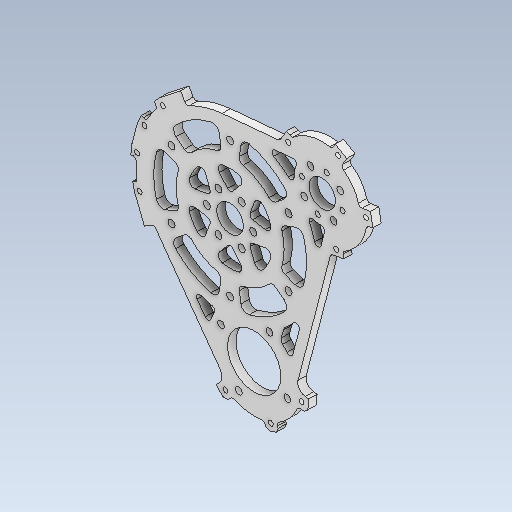
# Autodesk Inventor part: motor_h_1
Saved by Autodesk Inventor 2020 (Build 240168000, 168)
## iProperties
Created: 2020-07-14
Part Number: motor_h_1
Material: ABS Plastic
Document SubType Name: Modeling
Designer: psrobotics
Density: 1.06 g/cm^3
Appearance: Smooth - White
Author: psrobotics
Autodesk Inventor part; units mm, degrees
(part 1 of 3)
ref_plane "YZ Plane" through (0, 0, 0) normal (1, 0, 0) x (0, 1, 0)
ref_plane "XZ Plane" through (0, 0, 0) normal (0, 1, 0) x (-1, 0, 0)
ref_plane "XY Plane" through (0, 0, 0) normal (0, 0, 1) x (1, 0, 0)
sketch "Sketch1" plane through (0, 0, 0) normal (0, 0, 1) x (1, 0, 0)
  circle A0 centre (13.3039, -43.7854) radius 2.1 projected
  circle A1 centre (31.1494, -18.2994) radius 2.1 projected
  line L0 (8.7569, -41.0332) -> (9.9725, -47.9268) projected
  line L1 (12.5142, -47.4787) -> (9.9725, -47.9268) projected
  line L2 (17.8509, -46.5376) -> (12.5142, -47.4787) projected
  line L3 (17.2063, -42.8816) -> (17.8509, -46.5376) projected
  arc A2 (17.2063, -42.8816) -> (25.3756, -36.4162) centre (4.8498, -18.875) ccw projected
  arc A3 (25.3756, -36.4162) -> (28.3534, -32.1635) centre (4.8498, -18.875) ccw projected
  arc A4 (28.3534, -32.1635) -> (31.6348, -22.2755) centre (4.8498, -18.875) ccw projected
  line L4 (31.6348, -22.2755) -> (35.2909, -21.6308) projected
  line L5 (35.2909, -21.6308) -> (34.3498, -16.2941) projected
  line L6 (34.3498, -16.2941) -> (33.9017, -13.7524) projected
  line L7 (33.9017, -13.7524) -> (27.008, -14.9679) projected
  arc A5 (8.7569, -41.0332) -> (27.008, -14.9679) centre (4.8498, -18.875) ccw projected
  circle A6 centre (14.3857, 5.6417) radius 2.1 projected
  circle A7 centre (-15.6668, -2.4109) radius 2.1 projected
  line L8 (16.0998, 0.6106) -> (19.5998, 6.6727) projected
  line L9 (17.3647, 7.9632) -> (19.5998, 6.6727) projected
  line L10 (12.6716, 10.6727) -> (17.3647, 7.9632) projected
  line L11 (10.8154, 7.4577) -> (12.6716, 10.6727) projected
  arc A8 (10.8154, 7.4577) -> (0.4014, 7.756) centre (4.8498, -18.875) ccw projected
  arc A9 (0.4014, 7.756) -> (-4.6132, 6.4123) centre (4.8498, -18.875) ccw projected
  arc A10 (-4.6132, 6.4123) -> (-13.4829, 0.947) centre (4.8498, -18.875) ccw projected
  line L12 (-13.4829, 0.947) -> (-16.6979, 2.8032) projected
  line L13 (-16.6979, 2.8032) -> (-19.4075, -1.8899) projected
  line L14 (-19.4075, -1.8899) -> (-20.6979, -4.125) projected
  line L15 (-20.6979, -4.125) -> (-14.6357, -7.625) projected
  arc A11 (16.0998, 0.6106) -> (-14.6357, -7.625) centre (4.8498, -18.875) ccw projected
  circle A12 centre (-102.1649, -37.0532) radius 2.05 projected
  circle A13 centre (-91.1309, -21.0881) radius 2.05 projected
  circle A14 centre (-106.5395, -53.3794) radius 2.05 projected
  circle A15 centre (-104.9663, -72.7226) radius 2.05 projected
  line L16 (-76.835, -14.1568) -> (-80.3713, -8.0318) projected
  line L17 (-92.9509, -17.9357) -> (-80.3713, -8.0318) projected
  arc A16 (-92.9509, -17.9357) -> (-96.423, -21.7867) centre (-50.585, -59.6232) ccw projected
  line L18 (-95.6743, -22.4047) -> (-96.423, -21.7867) projected
  arc A17 (-95.3624, -25.1669) -> (-95.6743, -22.4047) centre (-96.9475, -23.9472) ccw projected
  arc A18 (-95.3624, -25.1669) -> (-100.1355, -32.4754) centre (-50.585, -59.6232) ccw projected
  arc A19 (-102.79, -33.3003) -> (-100.1355, -32.4754) centre (-101.8895, -31.5145) ccw projected
  line L19 (-103.9829, -32.6988) -> (-102.79, -33.3003) projected
  arc A20 (-103.9829, -32.6988) -> (-106.5047, -38.4279) centre (-50.585, -59.6232) ccw projected
  line L20 (-106.5047, -38.4279) -> (-109.6106, -50.019) projected
  arc A21 (-109.6106, -50.019) -> (-110.2911, -56.2415) centre (-50.585, -59.6232) ccw projected
  line L21 (-110.2911, -56.2415) -> (-108.9573, -56.317) projected
  arc A22 (-107.0709, -58.3586) -> (-108.9573, -56.317) centre (-109.0704, -58.3138) ccw projected
  arc A23 (-107.0709, -58.3586) -> (-106.5915, -67.0745) centre (-50.585, -59.6232) ccw projected
  arc A24 (-108.2427, -69.3107) -> (-106.5915, -67.0745) centre (-108.5741, -67.3383) ccw projected
  line L22 (-108.2427, -69.3107) -> (-109.2001, -69.4715) projected
  arc A25 (-109.2001, -69.4715) -> (-108.1187, -74.5427) centre (-50.585, -59.6232) ccw projected
  line L23 (-108.1187, -74.5427) -> (-102.1764, -89.4094) projected
  line L24 (-102.1764, -89.4094) -> (-96.0514, -85.8732) projected
  arc A26 (-76.835, -14.1568) -> (-96.0514, -85.8732) centre (-50.585, -59.6232) ccw projected
  line L25 (-21.6241, -154.5886) -> (-22.8103, -157.1563) projected
  line L26 (-21.6241, -154.5886) -> (-22.0027, -153.56) projected
  arc A27 (-21.1722, -151.1649) -> (-22.0027, -153.56) centre (-20.1257, -152.8693) ccw projected
  arc A28 (-21.1722, -151.1649) -> (-16.425, -147.5113) centre (-36.0848, -126.8778) ccw projected
  arc A29 (-16.425, -147.5113) -> (-12.2385, -142.4856) centre (-36.0848, -126.8778) ccw projected
  arc A30 (-12.2385, -142.4856) -> (-10.1895, -138.7808) centre (-36.0848, -126.8778) ccw projected
  arc A31 (-8.179, -137.6255) -> (-10.1895, -138.7808) centre (-8.3723, -139.6161) ccw projected
  line L27 (-8.179, -137.6255) -> (-6.0033, -137.8368) projected
  line L28 (-3.8193, -136.0394) -> (-6.0033, -137.8368) projected
  line L29 (-3.8193, -136.0394) -> (-3.2394, -130.0675) projected
  line L30 (-11.2019, -129.2943) -> (-3.2394, -130.0675) projected
  arc A32 (-53.4647, -144.8483) -> (-11.2019, -129.2943) centre (-36.0848, -126.8778) ccw projected
  line L31 (-53.4647, -144.8483) -> (-59.0263, -150.5988) projected
  line L32 (-59.0263, -150.5988) -> (-54.7134, -154.77) projected
  line L33 (-51.8854, -154.7228) -> (-54.7134, -154.77) projected
  line L34 (-51.8854, -154.7228) -> (-50.3657, -153.1515) projected
  arc A33 (-48.0859, -152.7278) -> (-50.3657, -153.1515) centre (-48.9281, -154.5419) ccw projected
  arc A34 (-48.0859, -152.7278) -> (-44.1241, -154.2204) centre (-36.0848, -126.8778) ccw projected
  arc A35 (-44.1241, -154.2204) -> (-37.6784, -155.3332) centre (-36.0848, -126.8778) ccw projected
  arc A36 (-37.6784, -155.3332) -> (-31.6953, -155.0377) centre (-36.0848, -126.8778) ccw projected
  arc A37 (-29.5104, -156.3231) -> (-31.6953, -155.0377) centre (-31.3873, -157.0139) ccw projected
  line L35 (-29.5104, -156.3231) -> (-29.1318, -157.3516) projected
  line L36 (-26.5641, -158.5378) -> (-29.1318, -157.3516) projected
  line L37 (-26.5641, -158.5378) -> (-22.8103, -157.1563) projected
  circle A38 centre (-53.3702, -150.5044) radius 2.05 projected
  circle A39 centre (-26.0687, -154.0932) radius 2.05 projected
  circle A40 centre (-7.6073, -133.6622) radius 2.05 projected
  circle A41 centre (4.8498, -18.875) radius 22.5
  circle A42 centre (-50.585, -59.6232) radius 52.5
  circle A43 centre (-36.0848, -126.8778) radius 25
  circle A44 centre (14.3857, 5.6417) radius 2.1 projected
  line L38 (-50.585, -59.6232) -> (-93.2051, -90.2791)
  line L39 (-36.0848, -126.8778) -> (-56.3801, -141.4758)
  line L40 (-56.3801, -141.4758) -> (-93.2051, -90.2791)
  line L41 (-50.585, -59.6232) -> (-55.4348, -7.3477)
  line L42 (-55.4348, -7.3477) -> (-20.6979, -4.125)
  line L43 (-11.2019, -129.2943) -> (9.9725, -47.9268)
  point P0 (0, 0)
  dimension "d2" = 50
  dimension "d0" = 45
  dimension "d1" = 105
  constraints: 12 end point, 3 coincident, 3 perpendicular, 2 centre point, 2 point on circle, 3 other
  measures "d0" diameter of A41
  measures "d1" diameter of A42
extrude "Extrusion4" add sketch "Sketch1" along normal blind 5 contours A0 | A1 | A5 L7 L6 L5 L4 A4 A3 A2 L3 L2 L1 L0 | A41 A42 A11 A5 | L0 L43 A43 A42 A41 | A42 A43 L38 L41 A41 | A41 A42 | L30 L29 L28 L27 A31 A30 A29 A28 A27 L26 L25 L37 L36 L35 A37 A36 A35 A34 A33 L34 L33 L32 L31 A32 | A32 A43 A42 | A42 L42 L15 A41 | A11 L15 L14 L13 L12 A10 A9 A8 L11 L10 L9 L8 | L41 L38 A42 A26 | A42 A43 | L40 A42 A43 | A26 L24 L23 A25 L22 A24 A23 A22 L21 A21 L20 A20 L19 A19 A18 A17 L18 A16 L17 L16 | A6 | A7 | A12 | A13 | A14 | A15 | A38 | A39 | A40
sketch "Sketch5" plane through (0, 0, 5) normal (0, 0, 1) x (1, 0, 0)
  circle A0 centre (-26.0687, -154.0932) radius 2.05 projected
  circle A1 centre (-53.3702, -150.5044) radius 2.05 projected
  circle A2 centre (-7.6073, -133.6622) radius 2.05 projected
  circle A3 centre (13.3039, -43.7854) radius 2.1 projected
  circle A4 centre (31.1494, -18.2994) radius 2.1 projected
  circle A5 centre (14.3857, 5.6417) radius 2.1 projected
  circle A6 centre (-15.6668, -2.4109) radius 2.1 projected
  circle A7 centre (-91.1309, -21.0881) radius 2.05 projected
  circle A8 centre (-102.1649, -37.0532) radius 2.05 projected
  circle A9 centre (-106.5395, -53.3794) radius 2.05 projected
  circle A10 centre (-104.9663, -72.7226) radius 2.05 projected
  point P0 (0, 0)
hole "Hole2" at (31.1494, -18.2994, 5) at (13.3039, -43.7854, 5) at (-15.6668, -2.4109, 5) at (14.3857, 5.6417, 5) at (-91.1309, -21.0881, 5) at (-102.1649, -37.0532, 5) at (-106.5395, -53.3794, 5) at (-104.9663, -72.7226, 5) at (-53.3702, -150.5044, 5) at (-26.0687, -154.0932, 5) at (-7.6073, -133.6622, 5) direction (0, 0, -1) diameter 3 depth 17
sketch "Sketch6" plane through (0, 0, 5) normal (0, 0, 1) x (1, 0, 0)
  circle A0 centre (-50.585, -59.6232) radius 50 projected
  circle A1 centre (-50.585, -59.6232) radius 5.075 projected
  circle A2 centre (4.8498, -18.875) radius 4.075 projected
  circle A3 centre (4.8498, -18.875) radius 8
  circle A4 centre (-50.585, -59.6232) radius 8
  point P0 (0, 0)
  dimension "d30" = 16
  dimension "d31" = 16
  constraints: 2 centre point, 2 coincident
  measures "d30" diameter of A3
  measures "d31" diameter of A4
extrude "Extrusion5" cut sketch "Sketch6" against normal blind 5 contours A1 | A2 | A3 | A4
sketch "Sketch7" plane through (0, 0, 5) normal (0, 0, 1) x (1, 0, 0)
  circle A0 centre (-36.0848, -126.8778) radius 17.5 projected
  circle A1 centre (-43.7823, -118.4013) radius 2.075 projected
  circle A2 centre (-28.3873, -135.3543) radius 2.075 projected
  circle A3 centre (-27.6083, -119.1803) radius 2.075 projected
  circle A4 centre (-44.5613, -134.5753) radius 2.075 projected
  circle A5 centre (-36.0848, -126.8778) radius 16
  point P0 (0, 0)
  dimension "d34" = 32
  constraints: 1 centre point, 1 coincident
  measures "d34" diameter of A5
extrude "Extrusion6" cut sketch "Sketch7" against normal blind 5 contours A1 | A2 | A3 | A4 | A5
fillet "Fillet6" radius 5 1 edges at (-11.2019, -129.2943, 2.5)
fillet "Fillet7" radius 6 1 edges at (-53.4647, -144.8483, 2.5)
sketch "Sketch8" plane through (0, 0, 5) normal (0, 0, 1) x (1, 0, 0)
  circle A0 centre (-36.0848, -126.8778) radius 16 projected
  circle A1 centre (-50.585, -59.6232) radius 8 projected
  circle A2 centre (4.8498, -18.875) radius 8 projected
  circle A3 centre (-26.0687, -154.0932) radius 1.5 projected
  circle A4 centre (-104.9663, -72.7226) radius 1.5 projected
  circle A5 centre (-102.1649, -37.0532) radius 1.5 projected
  circle A6 centre (14.3857, 5.6417) radius 1.5 projected
  circle A7 centre (13.3039, -43.7854) radius 1.5 projected
  circle A8 centre (31.1494, -18.2994) radius 1.5 projected
  circle A9 centre (-15.6668, -2.4109) radius 1.5 projected
  circle A10 centre (-91.1309, -21.0881) radius 1.5 projected
  circle A11 centre (-106.5395, -53.3794) radius 1.5 projected
  circle A12 centre (-53.3702, -150.5044) radius 1.5 projected
  circle A13 centre (-7.6073, -133.6622) radius 1.5 projected
  line L0 (-9.7265, -123.6247) -> (9.9725, -47.9268) projected
  line L1 (9.9725, -47.9268) -> (17.8509, -46.5376) projected
  line L2 (17.8509, -46.5376) -> (17.2063, -42.8816) projected
  arc A14 (17.2063, -42.8816) -> (31.6348, -22.2755) centre (4.8498, -18.875) ccw projected
  line L3 (31.6348, -22.2755) -> (35.2909, -21.6308) projected
  line L4 (35.2909, -21.6308) -> (33.9017, -13.7524) projected
  line L5 (33.9017, -13.7524) -> (27.008, -14.9679) projected
  arc A15 (27.008, -14.9679) -> (16.0998, 0.6106) centre (4.8498, -18.875) ccw projected
  line L6 (16.0998, 0.6106) -> (19.5998, 6.6727) projected
  line L7 (19.5998, 6.6727) -> (12.6716, 10.6727) projected
  line L8 (12.6716, 10.6727) -> (10.8154, 7.4577) projected
  arc A16 (10.8154, 7.4577) -> (-13.4829, 0.947) centre (4.8498, -18.875) ccw projected
  line L9 (-13.4829, 0.947) -> (-16.6979, 2.8032) projected
  line L10 (-16.6979, 2.8032) -> (-20.6979, -4.125) projected
  line L11 (-20.6979, -4.125) -> (-55.4348, -7.3477) projected
  arc A17 (-55.4348, -7.3477) -> (-76.835, -14.1568) centre (-50.585, -59.6232) ccw projected
  line L12 (-76.835, -14.1568) -> (-80.3713, -8.0318) projected
  line L13 (-80.3713, -8.0318) -> (-92.9509, -17.9357) projected
  arc A18 (-92.9509, -17.9357) -> (-96.423, -21.7867) centre (-50.585, -59.6232) ccw projected
  line L14 (-96.423, -21.7867) -> (-95.6743, -22.4047) projected
  arc A19 (-95.3624, -25.1669) -> (-95.6743, -22.4047) centre (-96.9475, -23.9472) ccw projected
  arc A20 (-95.3624, -25.1669) -> (-100.1355, -32.4754) centre (-50.585, -59.6232) ccw projected
  arc A21 (-102.79, -33.3003) -> (-100.1355, -32.4754) centre (-101.8895, -31.5145) ccw projected
  line L15 (-102.79, -33.3003) -> (-103.9829, -32.6988) projected
  arc A22 (-103.9829, -32.6988) -> (-106.5047, -38.4279) centre (-50.585, -59.6232) ccw projected
  line L16 (-106.5047, -38.4279) -> (-109.6106, -50.019) projected
  arc A23 (-109.6106, -50.019) -> (-110.2911, -56.2415) centre (-50.585, -59.6232) ccw projected
  line L17 (-110.2911, -56.2415) -> (-108.9573, -56.317) projected
  arc A24 (-107.0709, -58.3586) -> (-108.9573, -56.317) centre (-109.0704, -58.3138) ccw projected
  arc A25 (-107.0709, -58.3586) -> (-106.5915, -67.0745) centre (-50.585, -59.6232) ccw projected
  arc A26 (-108.2427, -69.3107) -> (-106.5915, -67.0745) centre (-108.5741, -67.3383) ccw projected
  line L18 (-108.2427, -69.3107) -> (-109.2001, -69.4715) projected
  arc A27 (-109.2001, -69.4715) -> (-108.1187, -74.5427) centre (-50.585, -59.6232) ccw projected
  line L19 (-108.1187, -74.5427) -> (-102.1764, -89.4094) projected
  line L20 (-102.1764, -89.4094) -> (-96.0514, -85.8732) projected
  arc A28 (-96.0514, -85.8732) -> (-93.2051, -90.2791) centre (-50.585, -59.6232) ccw projected
  line L21 (-93.2051, -90.2791) -> (-56.6733, -141.0681) projected
  arc A29 (-57.2313, -148.7428) -> (-56.6733, -141.0681) centre (-61.5442, -144.5716) ccw projected
  line L22 (-57.2313, -148.7428) -> (-59.0263, -150.5988) projected
  line L23 (-59.0263, -150.5988) -> (-54.7134, -154.77) projected
  line L24 (-54.7134, -154.77) -> (-51.8854, -154.7228) projected
  line L25 (-51.8854, -154.7228) -> (-50.3657, -153.1515) projected
  arc A30 (-48.0859, -152.7278) -> (-50.3657, -153.1515) centre (-48.9281, -154.5419) ccw projected
  arc A31 (-48.0859, -152.7278) -> (-31.6953, -155.0377) centre (-36.0848, -126.8778) ccw projected
  arc A32 (-29.5104, -156.3231) -> (-31.6953, -155.0377) centre (-31.3873, -157.0139) ccw projected
  line L26 (-29.5104, -156.3231) -> (-29.1318, -157.3516) projected
  line L27 (-29.1318, -157.3516) -> (-26.5641, -158.5378) projected
  line L28 (-26.5641, -158.5378) -> (-22.8103, -157.1563) projected
  line L29 (-22.8103, -157.1563) -> (-21.6241, -154.5886) projected
  line L30 (-21.6241, -154.5886) -> (-22.0027, -153.56) projected
  arc A33 (-21.1722, -151.1649) -> (-22.0027, -153.56) centre (-20.1257, -152.8693) ccw projected
  arc A34 (-21.1722, -151.1649) -> (-10.1895, -138.7808) centre (-36.0848, -126.8778) ccw projected
  arc A35 (-8.179, -137.6255) -> (-10.1895, -138.7808) centre (-8.3723, -139.6161) ccw projected
  line L31 (-8.179, -137.6255) -> (-6.0033, -137.8368) projected
  line L32 (-6.0033, -137.8368) -> (-3.8193, -136.0394) projected
  line L33 (-3.8193, -136.0394) -> (-3.2394, -130.0675) projected
  line L34 (-3.2394, -130.0675) -> (-5.371, -129.8605) projected
  arc A36 (-9.7265, -123.6247) -> (-5.371, -129.8605) centre (-4.8877, -124.8839) ccw projected
  circle A37 centre (-50.585, -59.6232) radius 15
  circle A38 centre (-50.585, -59.6232) radius 46
  circle A39 centre (-50.585, -59.6232) radius 32.5
  line L35 (-50.585, -59.6232) -> (3.2809, -73.6408)
  line L36 (-9.7265, -123.6247) -> (9.9725, -47.9268) projected
  line L37 (-50.585, -59.6232) -> (-38.3591, -103.9687)
  circle A40 centre (-50.585, -59.6232) radius 8 projected
  line L38 (-50.585, -59.6232) -> (-11.4, -83.7174)
  line L39 (-50.585, -59.6232) -> (-96.0514, -85.8732)
  line L40 (-50.585, -59.6232) -> (-86.3338, -88.5719)
  line L41 (-50.585, -59.6232) -> (-93.5297, -76.1081)
  line L42 (-50.585, -59.6232) -> (-93.5297, -43.1382)
  point P0 (0, 0)
  point P1 (-80.9264, -47.9762)
  point P2 (-80.9264, -71.2701)
  dimension "d39" = 30
  dimension "d40" = 92
  dimension "d41" = 65
  dimension "d42" = 60
  dimension "d43" = 17
  dimension "d44" = 9
  dimension "d45" = 9
  dimension "d46" = 42
  constraints: 14 end point, 5 point on circle, 3 centre point, 3 coincident, 1 perpendicular, 1 point on line
  measures "d39" diameter of A37
  measures "d40" diameter of A38
  measures "d41" diameter of A39
  measures "d42" angle of L35 L37
  measures "d43" angle of L35 L38
  measures "d44" angle of L39 L40
  measures "d45" angle of L39 L41
  measures "d46" angle of L41 L42
extrude "Extrusion7" cut sketch "Sketch8" against normal blind 10 contours A39 L41 A38 L42
pattern_circular "Circular Pattern1" count 6 over 360 about axis through (-50.585, -59.6232, 5) along (0, 0, -1) of "Extrusion7"
sketch "Sketch9" plane through (0, 0, 5) normal (0, 0, 1) x (1, 0, 0)
  arc A0 (-86.3338, -88.5719) -> (-57.781, -105.0568) centre (-50.585, -59.6232) ccw projected
  line L0 (-86.3338, -88.5719) -> (-75.8423, -80.0761) projected
  arc A1 (-75.8423, -80.0761) -> (-55.6692, -91.723) centre (-50.585, -59.6232) ccw projected
  line L1 (-55.6692, -91.723) -> (-57.781, -105.0568) projected
  arc A2 (-43.3891, -105.0568) -> (-14.8363, -88.5719) centre (-50.585, -59.6232) ccw projected
  line L2 (-43.3891, -105.0568) -> (-45.5009, -91.723) projected
  arc A3 (-45.5009, -91.723) -> (-25.3278, -80.0761) centre (-50.585, -59.6232) ccw projected
  line L3 (-25.3278, -80.0761) -> (-14.8363, -88.5719) projected
  arc A4 (-7.6403, -76.1081) -> (-7.6403, -43.1382) centre (-50.585, -59.6232) ccw projected
  line L4 (-7.6403, -76.1081) -> (-20.2437, -71.2701) projected
  arc A5 (-20.2437, -71.2701) -> (-20.2437, -47.9762) centre (-50.585, -59.6232) ccw projected
  line L5 (-20.2437, -47.9762) -> (-7.6403, -43.1382) projected
  arc A6 (-14.8363, -30.6744) -> (-43.3891, -14.1895) centre (-50.585, -59.6232) ccw projected
  line L6 (-14.8363, -30.6744) -> (-25.3278, -39.1703) projected
  arc A7 (-25.3278, -39.1703) -> (-45.5009, -27.5233) centre (-50.585, -59.6232) ccw projected
  line L7 (-45.5009, -27.5233) -> (-43.3891, -14.1895) projected
  arc A8 (-57.781, -14.1895) -> (-86.3338, -30.6744) centre (-50.585, -59.6232) ccw projected
  line L8 (-57.781, -14.1895) -> (-55.6692, -27.5233) projected
  arc A9 (-55.6692, -27.5233) -> (-75.8423, -39.1703) centre (-50.585, -59.6232) ccw projected
  line L9 (-75.8423, -39.1703) -> (-86.3338, -30.6744) projected
  arc A10 (-93.5297, -43.1382) -> (-93.5297, -76.1081) centre (-50.585, -59.6232) ccw projected
  line L10 (-93.5297, -43.1382) -> (-80.9264, -47.9762) projected
  arc A11 (-80.9264, -47.9762) -> (-80.9264, -71.2701) centre (-50.585, -59.6232) ccw projected
  line L11 (-80.9264, -71.2701) -> (-93.5297, -76.1081) projected
  circle A12 centre (-36.0848, -126.8778) radius 16 projected
  circle A13 centre (-50.585, -59.6232) radius 8 projected
  circle A14 centre (4.8498, -18.875) radius 8 projected
  circle A15 centre (-26.0687, -154.0932) radius 1.5 projected
  circle A16 centre (-104.9663, -72.7226) radius 1.5 projected
  circle A17 centre (-102.1649, -37.0532) radius 1.5 projected
  circle A18 centre (14.3857, 5.6417) radius 1.5 projected
  circle A19 centre (13.3039, -43.7854) radius 1.5 projected
  circle A20 centre (31.1494, -18.2994) radius 1.5 projected
  circle A21 centre (-15.6668, -2.4109) radius 1.5 projected
  circle A22 centre (-91.1309, -21.0881) radius 1.5 projected
  circle A23 centre (-106.5395, -53.3794) radius 1.5 projected
  circle A24 centre (-53.3702, -150.5044) radius 1.5 projected
  circle A25 centre (-7.6073, -133.6622) radius 1.5 projected
  line L12 (-9.7265, -123.6247) -> (9.9725, -47.9268) projected
  line L13 (9.9725, -47.9268) -> (17.8509, -46.5376) projected
  line L14 (17.8509, -46.5376) -> (17.2063, -42.8816) projected
  arc A26 (17.2063, -42.8816) -> (31.6348, -22.2755) centre (4.8498, -18.875) ccw projected
  line L15 (31.6348, -22.2755) -> (35.2909, -21.6308) projected
  line L16 (35.2909, -21.6308) -> (33.9017, -13.7524) projected
  line L17 (33.9017, -13.7524) -> (27.008, -14.9679) projected
  arc A27 (27.008, -14.9679) -> (16.0998, 0.6106) centre (4.8498, -18.875) ccw projected
  line L18 (16.0998, 0.6106) -> (19.5998, 6.6727) projected
  line L19 (19.5998, 6.6727) -> (12.6716, 10.6727) projected
  line L20 (12.6716, 10.6727) -> (10.8154, 7.4577) projected
  arc A28 (10.8154, 7.4577) -> (-13.4829, 0.947) centre (4.8498, -18.875) ccw projected
  line L21 (-13.4829, 0.947) -> (-16.6979, 2.8032) projected
  line L22 (-16.6979, 2.8032) -> (-20.6979, -4.125) projected
  line L23 (-20.6979, -4.125) -> (-55.4348, -7.3477) projected
  arc A29 (-55.4348, -7.3477) -> (-76.835, -14.1568) centre (-50.585, -59.6232) ccw projected
  line L24 (-76.835, -14.1568) -> (-80.3713, -8.0318) projected
  line L25 (-80.3713, -8.0318) -> (-92.9509, -17.9357) projected
  arc A30 (-92.9509, -17.9357) -> (-96.423, -21.7867) centre (-50.585, -59.6232) ccw projected
  line L26 (-96.423, -21.7867) -> (-95.6743, -22.4047) projected
  arc A31 (-95.3624, -25.1669) -> (-95.6743, -22.4047) centre (-96.9475, -23.9472) ccw projected
  arc A32 (-95.3624, -25.1669) -> (-100.1355, -32.4754) centre (-50.585, -59.6232) ccw projected
  arc A33 (-102.79, -33.3003) -> (-100.1355, -32.4754) centre (-101.8895, -31.5145) ccw projected
  line L27 (-102.79, -33.3003) -> (-103.9829, -32.6988) projected
  arc A34 (-103.9829, -32.6988) -> (-106.5047, -38.4279) centre (-50.585, -59.6232) ccw projected
  line L28 (-106.5047, -38.4279) -> (-109.6106, -50.019) projected
  arc A35 (-109.6106, -50.019) -> (-110.2911, -56.2415) centre (-50.585, -59.6232) ccw projected
  line L29 (-110.2911, -56.2415) -> (-108.9573, -56.317) projected
  arc A36 (-107.0709, -58.3586) -> (-108.9573, -56.317) centre (-109.0704, -58.3138) ccw projected
  arc A37 (-107.0709, -58.3586) -> (-106.5915, -67.0745) centre (-50.585, -59.6232) ccw projected
  arc A38 (-108.2427, -69.3107) -> (-106.5915, -67.0745) centre (-108.5741, -67.3383) ccw projected
  line L30 (-108.2427, -69.3107) -> (-109.2001, -69.4715) projected
  arc A39 (-109.2001, -69.4715) -> (-108.1187, -74.5427) centre (-50.585, -59.6232) ccw projected
  line L31 (-108.1187, -74.5427) -> (-102.1764, -89.4094) projected
  line L32 (-102.1764, -89.4094) -> (-96.0514, -85.8732) projected
  arc A40 (-96.0514, -85.8732) -> (-93.2051, -90.2791) centre (-50.585, -59.6232) ccw projected
  line L33 (-93.2051, -90.2791) -> (-56.6733, -141.0681) projected
  arc A41 (-57.2313, -148.7428) -> (-56.6733, -141.0681) centre (-61.5442, -144.5716) ccw projected
  line L34 (-57.2313, -148.7428) -> (-59.0263, -150.5988) projected
  line L35 (-59.0263, -150.5988) -> (-54.7134, -154.77) projected
  line L36 (-54.7134, -154.77) -> (-51.8854, -154.7228) projected
  line L37 (-51.8854, -154.7228) -> (-50.3657, -153.1515) projected
  arc A42 (-48.0859, -152.7278) -> (-50.3657, -153.1515) centre (-48.9281, -154.5419) ccw projected
  arc A43 (-48.0859, -152.7278) -> (-31.6953, -155.0377) centre (-36.0848, -126.8778) ccw projected
  arc A44 (-29.5104, -156.3231) -> (-31.6953, -155.0377) centre (-31.3873, -157.0139) ccw projected
  line L38 (-29.5104, -156.3231) -> (-29.1318, -157.3516) projected
  line L39 (-29.1318, -157.3516) -> (-26.5641, -158.5378) projected
  line L40 (-26.5641, -158.5378) -> (-22.8103, -157.1563) projected
  line L41 (-22.8103, -157.1563) -> (-21.6241, -154.5886) projected
  line L42 (-21.6241, -154.5886) -> (-22.0027, -153.56) projected
  arc A45 (-21.1722, -151.1649) -> (-22.0027, -153.56) centre (-20.1257, -152.8693) ccw projected
  arc A46 (-21.1722, -151.1649) -> (-10.1895, -138.7808) centre (-36.0848, -126.8778) ccw projected
  arc A47 (-8.179, -137.6255) -> (-10.1895, -138.7808) centre (-8.3723, -139.6161) ccw projected
  line L43 (-8.179, -137.6255) -> (-6.0033, -137.8368) projected
  line L44 (-6.0033, -137.8368) -> (-3.8193, -136.0394) projected
  line L45 (-3.8193, -136.0394) -> (-3.2394, -130.0675) projected
  line L46 (-3.2394, -130.0675) -> (-5.371, -129.8605) projected
  arc A48 (-9.7265, -123.6247) -> (-5.371, -129.8605) centre (-4.8877, -124.8839) ccw projected
  circle A49 centre (-50.585, -59.6232) radius 8 projected
  circle A50 centre (-50.585, -59.6232) radius 13
  circle A51 centre (-50.585, -59.6232) radius 26
  line L47 (-25.3278, -39.1703) -> (-20.2437, -47.9762)
  line L48 (-50.585, -59.6232) -> (-22.7857, -43.5732)
  line L49 (-39.3267, -53.1232) -> (-24.8875, -55.6692)
  line L50 (-39.3267, -53.1232) -> (-34.312, -39.3454)
  point P0 (0, 0)
  dimension "d52" = 26
  dimension "d53" = 52
  dimension "d54" = 40
  dimension "d55" = 40
  constraints: 8 end point, 2 coincident, 2 point on circle, 1 centre point, 1 midpoint, 1 point on line, 3 other
  measures "d53" diameter of A51
  measures "d54" angle of L48 L49
  measures "d55" angle of L48 L50
extrude "Extrusion8" cut sketch "Sketch9" against normal blind 10 contours L50 A51 L48 | L48 A51 L49
pattern_circular "Circular Pattern2" count 6 over 360 about axis through (-50.585, -59.6232, 5) along (0, 0, -1) of "Extrusion8"
fillet "Fillet8" radius 3 2 edges at (-34.312, -39.3454, 2.5) (-24.8875, -55.6692, 2.5)
fillet "Fillet9" radius 2 1 edges at (-39.3267, -53.1232, 2.5)
pattern_circular "Circular Pattern3" count 6 over 360 about axis through (-50.585, -59.6232, 5) along (0, 0, -1) of "Fillet8", "Fillet9"
fillet "Fillet10" radius 3 2 edges at (-45.5009, -27.5233, 2.5) (-25.3278, -39.1703, 2.5)
fillet "Fillet11" radius 4 2 edges at (-43.3891, -14.1895, 2.5) (-14.8363, -30.6744, 2.5)
pattern_circular "Circular Pattern4" count 6 over 360 about axis through (-50.585, -59.6232, 5) along (0, 0, -1) of "Fillet10", "Fillet11"
sketch "Sketch10" plane through (0, 0, 5) normal (0, 0, 1) x (1, 0, 0)
  line L0 (-44.13, -38.9303) -> (-49.053, -44.7973) projected
  arc A0 (-52.1171, -44.7973) -> (-49.053, -44.7973) centre (-50.585, -43.5117) ccw projected
  line L1 (-52.1171, -44.7973) -> (-57.0401, -38.9303) projected
  arc A1 (-55.2842, -34.0514) -> (-57.0401, -38.9303) centre (-54.742, -37.0019) ccw projected
  arc A2 (-45.8859, -34.0514) -> (-55.2842, -34.0514) centre (-50.585, -59.6232) ccw projected
  arc A3 (-44.13, -38.9303) -> (-45.8859, -34.0514) centre (-46.4281, -37.0019) ccw projected
  line L2 (-65.2781, -43.6865) -> (-62.6586, -50.8834) projected
  arc A4 (-64.1907, -53.5371) -> (-62.6586, -50.8834) centre (-64.538, -51.5674) ccw projected
  line L3 (-64.1907, -53.5371) -> (-71.7331, -54.867) projected
  arc A5 (-75.0805, -50.9068) -> (-71.7331, -54.867) centre (-72.2541, -51.9126) ccw projected
  arc A6 (-70.3813, -42.7677) -> (-75.0805, -50.9068) centre (-50.585, -59.6232) ccw projected
  arc A7 (-65.2781, -43.6865) -> (-70.3813, -42.7677) centre (-68.0971, -44.7125) ccw projected
  line L4 (-71.7331, -64.3793) -> (-64.1907, -65.7093) projected
  arc A8 (-62.6586, -68.3629) -> (-64.1907, -65.7093) centre (-64.538, -67.6789) ccw projected
  line L5 (-62.6586, -68.3629) -> (-65.2781, -75.5599) projected
  arc A9 (-70.3813, -76.4787) -> (-65.2781, -75.5599) centre (-68.0971, -74.5338) ccw projected
  arc A10 (-75.0805, -68.3395) -> (-70.3813, -76.4787) centre (-50.585, -59.6232) ccw projected
  arc A11 (-71.7331, -64.3793) -> (-75.0805, -68.3395) centre (-72.2541, -67.3338) ccw projected
  line L6 (-57.0401, -80.316) -> (-52.1171, -74.449) projected
  arc A12 (-49.053, -74.449) -> (-52.1171, -74.449) centre (-50.585, -75.7346) ccw projected
  line L7 (-49.053, -74.449) -> (-44.13, -80.316) projected
  arc A13 (-45.8859, -85.195) -> (-44.13, -80.316) centre (-46.4281, -82.2444) ccw projected
  arc A14 (-55.2842, -85.195) -> (-45.8859, -85.195) centre (-50.585, -59.6232) ccw projected
  arc A15 (-57.0401, -80.316) -> (-55.2842, -85.195) centre (-54.742, -82.2444) ccw projected
  line L8 (-35.892, -75.5599) -> (-38.5115, -68.3629) projected
  arc A16 (-36.9794, -65.7093) -> (-38.5115, -68.3629) centre (-36.6321, -67.6789) ccw projected
  line L9 (-36.9794, -65.7093) -> (-29.437, -64.3793) projected
  arc A17 (-26.0896, -68.3395) -> (-29.437, -64.3793) centre (-28.916, -67.3338) ccw projected
  arc A18 (-30.7888, -76.4787) -> (-26.0896, -68.3395) centre (-50.585, -59.6232) ccw projected
  arc A19 (-35.892, -75.5599) -> (-30.7888, -76.4787) centre (-33.073, -74.5338) ccw projected
  line L10 (-29.437, -54.867) -> (-36.9794, -53.5371) projected
  arc A20 (-38.5115, -50.8834) -> (-36.9794, -53.5371) centre (-36.6321, -51.5674) ccw projected
  line L11 (-38.5115, -50.8834) -> (-35.892, -43.6865) projected
  arc A21 (-30.7888, -42.7677) -> (-35.892, -43.6865) centre (-33.073, -44.7125) ccw projected
  arc A22 (-26.0896, -50.9068) -> (-30.7888, -42.7677) centre (-50.585, -59.6232) ccw projected
  arc A23 (-29.437, -54.867) -> (-26.0896, -50.9068) centre (-28.916, -51.9126) ccw projected
  arc A24 (-83.4142, -91.845) -> (-62.0753, -104.165) centre (-50.585, -59.6232) ccw projected
  arc A25 (-83.0768, -85.9345) -> (-83.4142, -91.845) centre (-80.5595, -89.0431) ccw projected
  line L12 (-83.0768, -85.9345) -> (-78.075, -81.8841) projected
  arc A26 (-74.0235, -82.1373) -> (-78.075, -81.8841) centre (-76.1871, -84.2156) ccw projected
  arc A27 (-74.0235, -82.1373) -> (-58.3636, -91.1786) centre (-50.585, -59.6232) ccw projected
  arc A28 (-56.1186, -94.5607) -> (-58.3636, -91.1786) centre (-59.0817, -94.0914) ccw projected
  line L13 (-56.1186, -94.5607) -> (-57.1254, -100.9175) projected
  arc A29 (-62.0753, -104.165) -> (-57.1254, -100.9175) centre (-61.0762, -100.2918) ccw projected
  arc A30 (-39.0948, -104.165) -> (-17.7559, -91.845) centre (-50.585, -59.6232) ccw projected
  arc A31 (-44.0447, -100.9175) -> (-39.0948, -104.165) centre (-40.0939, -100.2918) ccw projected
  line L14 (-44.0447, -100.9175) -> (-45.0515, -94.5607) projected
  arc A32 (-42.8065, -91.1786) -> (-45.0515, -94.5607) centre (-42.0884, -94.0914) ccw projected
  arc A33 (-42.8065, -91.1786) -> (-27.1466, -82.1373) centre (-50.585, -59.6232) ccw projected
  arc A34 (-23.0951, -81.8841) -> (-27.1466, -82.1373) centre (-24.983, -84.2156) ccw projected
  line L15 (-23.0951, -81.8841) -> (-18.0933, -85.9345) projected
  arc A35 (-17.7559, -91.845) -> (-18.0933, -85.9345) centre (-20.6106, -89.0431) ccw projected
  arc A36 (-6.2656, -71.9432) -> (-6.2656, -47.3031) centre (-50.585, -59.6232) ccw projected
  arc A37 (-11.5529, -74.6062) -> (-6.2656, -71.9432) centre (-10.1194, -70.8719) ccw projected
  line L16 (-11.5529, -74.6062) -> (-17.5615, -72.2997) projected
  arc A38 (-19.368, -68.6644) -> (-17.5615, -72.2997) centre (-16.4864, -69.499) ccw projected
  arc A39 (-19.368, -68.6644) -> (-19.368, -50.5819) centre (-50.585, -59.6232) ccw projected
  arc A40 (-17.5615, -46.9466) -> (-19.368, -50.5819) centre (-16.4864, -49.7474) ccw projected
  line L17 (-17.5615, -46.9466) -> (-11.5529, -44.6401) projected
  arc A41 (-6.2656, -47.3031) -> (-11.5529, -44.6401) centre (-10.1194, -48.3745) ccw projected
  arc A42 (-17.7559, -27.4014) -> (-39.0948, -15.0814) centre (-50.585, -59.6232) ccw projected
  arc A43 (-18.0933, -33.3119) -> (-17.7559, -27.4014) centre (-20.6106, -30.2033) ccw projected
  line L18 (-18.0933, -33.3119) -> (-23.0951, -37.3622) projected
  arc A44 (-27.1466, -37.109) -> (-23.0951, -37.3622) centre (-24.983, -35.0308) ccw projected
  arc A45 (-27.1466, -37.109) -> (-42.8065, -28.0678) centre (-50.585, -59.6232) ccw projected
  arc A46 (-45.0515, -24.6857) -> (-42.8065, -28.0678) centre (-42.0884, -25.155) ccw projected
  line L19 (-45.0515, -24.6857) -> (-44.0447, -18.3288) projected
  arc A47 (-39.0948, -15.0814) -> (-44.0447, -18.3288) centre (-40.0939, -18.9546) ccw projected
  arc A48 (-62.0753, -15.0814) -> (-83.4142, -27.4014) centre (-50.585, -59.6232) ccw projected
  arc A49 (-57.1254, -18.3288) -> (-62.0753, -15.0814) centre (-61.0762, -18.9546) ccw projected
  line L20 (-57.1254, -18.3288) -> (-56.1186, -24.6857) projected
  arc A50 (-58.3636, -28.0678) -> (-56.1186, -24.6857) centre (-59.0817, -25.155) ccw projected
  arc A51 (-58.3636, -28.0678) -> (-74.0235, -37.109) centre (-50.585, -59.6232) ccw projected
  arc A52 (-78.075, -37.3622) -> (-74.0235, -37.109) centre (-76.1871, -35.0308) ccw projected
  line L21 (-78.075, -37.3622) -> (-83.0768, -33.3119) projected
  arc A53 (-83.4142, -27.4014) -> (-83.0768, -33.3119) centre (-80.5595, -30.2033) ccw projected
  arc A54 (-94.9045, -47.3031) -> (-94.9045, -71.9432) centre (-50.585, -59.6232) ccw projected
  arc A55 (-89.6172, -44.6401) -> (-94.9045, -47.3031) centre (-91.0507, -48.3745) ccw projected
  line L22 (-89.6172, -44.6401) -> (-83.6086, -46.9466) projected
  arc A56 (-81.8021, -50.5819) -> (-83.6086, -46.9466) centre (-84.6837, -49.7474) ccw projected
  arc A57 (-81.8021, -50.5819) -> (-81.8021, -68.6644) centre (-50.585, -59.6232) ccw projected
  arc A58 (-83.6086, -72.2997) -> (-81.8021, -68.6644) centre (-84.6837, -69.499) ccw projected
  line L23 (-83.6086, -72.2997) -> (-89.6172, -74.6062) projected
  arc A59 (-94.9045, -71.9432) -> (-89.6172, -74.6062) centre (-91.0507, -70.8719) ccw projected
  circle A60 centre (-36.0848, -126.8778) radius 16 projected
  circle A61 centre (-50.585, -59.6232) radius 8 projected
  circle A62 centre (4.8498, -18.875) radius 8 projected
  circle A63 centre (-26.0687, -154.0932) radius 1.5 projected
  circle A64 centre (-104.9663, -72.7226) radius 1.5 projected
  circle A65 centre (-102.1649, -37.0532) radius 1.5 projected
  circle A66 centre (14.3857, 5.6417) radius 1.5 projected
  circle A67 centre (13.3039, -43.7854) radius 1.5 projected
  circle A68 centre (31.1494, -18.2994) radius 1.5 projected
  circle A69 centre (-15.6668, -2.4109) radius 1.5 projected
  circle A70 centre (-91.1309, -21.0881) radius 1.5 projected
  circle A71 centre (-106.5395, -53.3794) radius 1.5 projected
  circle A72 centre (-53.3702, -150.5044) radius 1.5 projected
  circle A73 centre (-7.6073, -133.6622) radius 1.5 projected
  line L24 (-9.7265, -123.6247) -> (9.9725, -47.9268) projected
  line L25 (9.9725, -47.9268) -> (17.8509, -46.5376) projected
  line L26 (17.8509, -46.5376) -> (17.2063, -42.8816) projected
  arc A74 (17.2063, -42.8816) -> (31.6348, -22.2755) centre (4.8498, -18.875) ccw projected
  line L27 (31.6348, -22.2755) -> (35.2909, -21.6308) projected
  line L28 (35.2909, -21.6308) -> (33.9017, -13.7524) projected
  line L29 (33.9017, -13.7524) -> (27.008, -14.9679) projected
  arc A75 (27.008, -14.9679) -> (16.0998, 0.6106) centre (4.8498, -18.875) ccw projected
  line L30 (16.0998, 0.6106) -> (19.5998, 6.6727) projected
  line L31 (19.5998, 6.6727) -> (12.6716, 10.6727) projected
  line L32 (12.6716, 10.6727) -> (10.8154, 7.4577) projected
  arc A76 (10.8154, 7.4577) -> (-13.4829, 0.947) centre (4.8498, -18.875) ccw projected
  line L33 (-13.4829, 0.947) -> (-16.6979, 2.8032) projected
  line L34 (-16.6979, 2.8032) -> (-20.6979, -4.125) projected
  line L35 (-20.6979, -4.125) -> (-55.4348, -7.3477) projected
  arc A77 (-55.4348, -7.3477) -> (-76.835, -14.1568) centre (-50.585, -59.6232) ccw projected
  line L36 (-76.835, -14.1568) -> (-80.3713, -8.0318) projected
  line L37 (-80.3713, -8.0318) -> (-92.9509, -17.9357) projected
  arc A78 (-92.9509, -17.9357) -> (-96.423, -21.7867) centre (-50.585, -59.6232) ccw projected
  line L38 (-96.423, -21.7867) -> (-95.6743, -22.4047) projected
  arc A79 (-95.3624, -25.1669) -> (-95.6743, -22.4047) centre (-96.9475, -23.9472) ccw projected
  arc A80 (-95.3624, -25.1669) -> (-100.1355, -32.4754) centre (-50.585, -59.6232) ccw projected
  arc A81 (-102.79, -33.3003) -> (-100.1355, -32.4754) centre (-101.8895, -31.5145) ccw projected
  line L39 (-102.79, -33.3003) -> (-103.9829, -32.6988) projected
  arc A82 (-103.9829, -32.6988) -> (-106.5047, -38.4279) centre (-50.585, -59.6232) ccw projected
  line L40 (-106.5047, -38.4279) -> (-109.6106, -50.019) projected
  arc A83 (-109.6106, -50.019) -> (-110.2911, -56.2415) centre (-50.585, -59.6232) ccw projected
  line L41 (-110.2911, -56.2415) -> (-108.9573, -56.317) projected
  arc A84 (-107.0709, -58.3586) -> (-108.9573, -56.317) centre (-109.0704, -58.3138) ccw projected
  arc A85 (-107.0709, -58.3586) -> (-106.5915, -67.0745) centre (-50.585, -59.6232) ccw projected
  arc A86 (-108.2427, -69.3107) -> (-106.5915, -67.0745) centre (-108.5741, -67.3383) ccw projected
  line L42 (-108.2427, -69.3107) -> (-109.2001, -69.4715) projected
  arc A87 (-109.2001, -69.4715) -> (-108.1187, -74.5427) centre (-50.585, -59.6232) ccw projected
  line L43 (-108.1187, -74.5427) -> (-102.1764, -89.4094) projected
  line L44 (-102.1764, -89.4094) -> (-96.0514, -85.8732) projected
  arc A88 (-96.0514, -85.8732) -> (-93.2051, -90.2791) centre (-50.585, -59.6232) ccw projected
  line L45 (-93.2051, -90.2791) -> (-56.6733, -141.0681) projected
  arc A89 (-57.2313, -148.7428) -> (-56.6733, -141.0681) centre (-61.5442, -144.5716) ccw projected
  line L46 (-57.2313, -148.7428) -> (-59.0263, -150.5988) projected
  line L47 (-59.0263, -150.5988) -> (-54.7134, -154.77) projected
  line L48 (-54.7134, -154.77) -> (-51.8854, -154.7228) projected
  line L49 (-51.8854, -154.7228) -> (-50.3657, -153.1515) projected
  arc A90 (-48.0859, -152.7278) -> (-50.3657, -153.1515) centre (-48.9281, -154.5419) ccw projected
  arc A91 (-48.0859, -152.7278) -> (-31.6953, -155.0377) centre (-36.0848, -126.8778) ccw projected
  arc A92 (-29.5104, -156.3231) -> (-31.6953, -155.0377) centre (-31.3873, -157.0139) ccw projected
  line L50 (-29.5104, -156.3231) -> (-29.1318, -157.3516) projected
  line L51 (-29.1318, -157.3516) -> (-26.5641, -158.5378) projected
  line L52 (-26.5641, -158.5378) -> (-22.8103, -157.1563) projected
  line L53 (-22.8103, -157.1563) -> (-21.6241, -154.5886) projected
  line L54 (-21.6241, -154.5886) -> (-22.0027, -153.56) projected
  arc A93 (-21.1722, -151.1649) -> (-22.0027, -153.56) centre (-20.1257, -152.8693) ccw projected
  arc A94 (-21.1722, -151.1649) -> (-10.1895, -138.7808) centre (-36.0848, -126.8778) ccw projected
  arc A95 (-8.179, -137.6255) -> (-10.1895, -138.7808) centre (-8.3723, -139.6161) ccw projected
  line L55 (-8.179, -137.6255) -> (-6.0033, -137.8368) projected
  line L56 (-6.0033, -137.8368) -> (-3.8193, -136.0394) projected
  line L57 (-3.8193, -136.0394) -> (-3.2394, -130.0675) projected
  line L58 (-3.2394, -130.0675) -> (-5.371, -129.8605) projected
  arc A96 (-9.7265, -123.6247) -> (-5.371, -129.8605) centre (-4.8877, -124.8839) ccw projected
  line L59 (-36.6321, -51.5674) -> (-36.6321, -67.6789)
  circle A97 centre (-36.6321, -59.6232) radius 2.1
  point P0 (0, 0)
  dimension "d71" = 4.2
  constraints: 2 end point, 1 centre point, 1 midpoint, 1 vertical
  measures "d71" diameter of A97
extrude "Extrusion9" cut sketch "Sketch10" against normal blind 10 contours A97 L59 | L59 A97
sketch "Sketch11" plane through (0, 0, 5) normal (0, 0, 1) x (1, 0, 0)
  circle A0 centre (-36.6321, -59.6232) radius 2.1 projected
  line L0 (-44.13, -38.9303) -> (-49.053, -44.7973) projected
  arc A1 (-52.1171, -44.7973) -> (-49.053, -44.7973) centre (-50.585, -43.5117) ccw projected
  line L1 (-52.1171, -44.7973) -> (-57.0401, -38.9303) projected
  arc A2 (-55.2842, -34.0514) -> (-57.0401, -38.9303) centre (-54.742, -37.0019) ccw projected
  arc A3 (-45.8859, -34.0514) -> (-55.2842, -34.0514) centre (-50.585, -59.6232) ccw projected
  arc A4 (-44.13, -38.9303) -> (-45.8859, -34.0514) centre (-46.4281, -37.0019) ccw projected
  line L2 (-65.2781, -43.6865) -> (-62.6586, -50.8834) projected
  arc A5 (-64.1907, -53.5371) -> (-62.6586, -50.8834) centre (-64.538, -51.5674) ccw projected
  line L3 (-64.1907, -53.5371) -> (-71.7331, -54.867) projected
  arc A6 (-75.0805, -50.9068) -> (-71.7331, -54.867) centre (-72.2541, -51.9126) ccw projected
  arc A7 (-70.3813, -42.7677) -> (-75.0805, -50.9068) centre (-50.585, -59.6232) ccw projected
  arc A8 (-65.2781, -43.6865) -> (-70.3813, -42.7677) centre (-68.0971, -44.7125) ccw projected
  line L4 (-71.7331, -64.3793) -> (-64.1907, -65.7093) projected
  arc A9 (-62.6586, -68.3629) -> (-64.1907, -65.7093) centre (-64.538, -67.6789) ccw projected
  line L5 (-62.6586, -68.3629) -> (-65.2781, -75.5599) projected
  arc A10 (-70.3813, -76.4787) -> (-65.2781, -75.5599) centre (-68.0971, -74.5338) ccw projected
  arc A11 (-75.0805, -68.3395) -> (-70.3813, -76.4787) centre (-50.585, -59.6232) ccw projected
  arc A12 (-71.7331, -64.3793) -> (-75.0805, -68.3395) centre (-72.2541, -67.3338) ccw projected
  line L6 (-57.0401, -80.316) -> (-52.1171, -74.449) projected
  arc A13 (-49.053, -74.449) -> (-52.1171, -74.449) centre (-50.585, -75.7346) ccw projected
  line L7 (-49.053, -74.449) -> (-44.13, -80.316) projected
  arc A14 (-45.8859, -85.195) -> (-44.13, -80.316) centre (-46.4281, -82.2444) ccw projected
  arc A15 (-55.2842, -85.195) -> (-45.8859, -85.195) centre (-50.585, -59.6232) ccw projected
  arc A16 (-57.0401, -80.316) -> (-55.2842, -85.195) centre (-54.742, -82.2444) ccw projected
  line L8 (-35.892, -75.5599) -> (-38.5115, -68.3629) projected
  arc A17 (-36.9794, -65.7093) -> (-38.5115, -68.3629) centre (-36.6321, -67.6789) ccw projected
  line L9 (-36.9794, -65.7093) -> (-29.437, -64.3793) projected
  arc A18 (-26.0896, -68.3395) -> (-29.437, -64.3793) centre (-28.916, -67.3338) ccw projected
  arc A19 (-30.7888, -76.4787) -> (-26.0896, -68.3395) centre (-50.585, -59.6232) ccw projected
  arc A20 (-35.892, -75.5599) -> (-30.7888, -76.4787) centre (-33.073, -74.5338) ccw projected
  line L10 (-29.437, -54.867) -> (-36.9794, -53.5371) projected
  arc A21 (-38.5115, -50.8834) -> (-36.9794, -53.5371) centre (-36.6321, -51.5674) ccw projected
  line L11 (-38.5115, -50.8834) -> (-35.892, -43.6865) projected
  arc A22 (-30.7888, -42.7677) -> (-35.892, -43.6865) centre (-33.073, -44.7125) ccw projected
  arc A23 (-26.0896, -50.9068) -> (-30.7888, -42.7677) centre (-50.585, -59.6232) ccw projected
  arc A24 (-29.437, -54.867) -> (-26.0896, -50.9068) centre (-28.916, -51.9126) ccw projected
  arc A25 (-83.4142, -91.845) -> (-62.0753, -104.165) centre (-50.585, -59.6232) ccw projected
  arc A26 (-83.0768, -85.9345) -> (-83.4142, -91.845) centre (-80.5595, -89.0431) ccw projected
  line L12 (-83.0768, -85.9345) -> (-78.075, -81.8841) projected
  arc A27 (-74.0235, -82.1373) -> (-78.075, -81.8841) centre (-76.1871, -84.2156) ccw projected
  arc A28 (-74.0235, -82.1373) -> (-58.3636, -91.1786) centre (-50.585, -59.6232) ccw projected
  arc A29 (-56.1186, -94.5607) -> (-58.3636, -91.1786) centre (-59.0817, -94.0914) ccw projected
  line L13 (-56.1186, -94.5607) -> (-57.1254, -100.9175) projected
  arc A30 (-62.0753, -104.165) -> (-57.1254, -100.9175) centre (-61.0762, -100.2918) ccw projected
  arc A31 (-39.0948, -104.165) -> (-17.7559, -91.845) centre (-50.585, -59.6232) ccw projected
  arc A32 (-44.0447, -100.9175) -> (-39.0948, -104.165) centre (-40.0939, -100.2918) ccw projected
  line L14 (-44.0447, -100.9175) -> (-45.0515, -94.5607) projected
  arc A33 (-42.8065, -91.1786) -> (-45.0515, -94.5607) centre (-42.0884, -94.0914) ccw projected
  arc A34 (-42.8065, -91.1786) -> (-27.1466, -82.1373) centre (-50.585, -59.6232) ccw projected
  arc A35 (-23.0951, -81.8841) -> (-27.1466, -82.1373) centre (-24.983, -84.2156) ccw projected
  line L15 (-23.0951, -81.8841) -> (-18.0933, -85.9345) projected
  arc A36 (-17.7559, -91.845) -> (-18.0933, -85.9345) centre (-20.6106, -89.0431) ccw projected
  arc A37 (-6.2656, -71.9432) -> (-6.2656, -47.3031) centre (-50.585, -59.6232) ccw projected
  arc A38 (-11.5529, -74.6062) -> (-6.2656, -71.9432) centre (-10.1194, -70.8719) ccw projected
  line L16 (-11.5529, -74.6062) -> (-17.5615, -72.2997) projected
  arc A39 (-19.368, -68.6644) -> (-17.5615, -72.2997) centre (-16.4864, -69.499) ccw projected
  arc A40 (-19.368, -68.6644) -> (-19.368, -50.5819) centre (-50.585, -59.6232) ccw projected
  arc A41 (-17.5615, -46.9466) -> (-19.368, -50.5819) centre (-16.4864, -49.7474) ccw projected
  line L17 (-17.5615, -46.9466) -> (-11.5529, -44.6401) projected
  arc A42 (-6.2656, -47.3031) -> (-11.5529, -44.6401) centre (-10.1194, -48.3745) ccw projected
  arc A43 (-17.7559, -27.4014) -> (-39.0948, -15.0814) centre (-50.585, -59.6232) ccw projected
  arc A44 (-18.0933, -33.3119) -> (-17.7559, -27.4014) centre (-20.6106, -30.2033) ccw projected
  line L18 (-18.0933, -33.3119) -> (-23.0951, -37.3622) projected
  arc A45 (-27.1466, -37.109) -> (-23.0951, -37.3622) centre (-24.983, -35.0308) ccw projected
  arc A46 (-27.1466, -37.109) -> (-42.8065, -28.0678) centre (-50.585, -59.6232) ccw projected
  arc A47 (-45.0515, -24.6857) -> (-42.8065, -28.0678) centre (-42.0884, -25.155) ccw projected
  line L19 (-45.0515, -24.6857) -> (-44.0447, -18.3288) projected
  arc A48 (-39.0948, -15.0814) -> (-44.0447, -18.3288) centre (-40.0939, -18.9546) ccw projected
  arc A49 (-62.0753, -15.0814) -> (-83.4142, -27.4014) centre (-50.585, -59.6232) ccw projected
  arc A50 (-57.1254, -18.3288) -> (-62.0753, -15.0814) centre (-61.0762, -18.9546) ccw projected
  line L20 (-57.1254, -18.3288) -> (-56.1186, -24.6857) projected
  arc A51 (-58.3636, -28.0678) -> (-56.1186, -24.6857) centre (-59.0817, -25.155) ccw projected
  arc A52 (-58.3636, -28.0678) -> (-74.0235, -37.109) centre (-50.585, -59.6232) ccw projected
  arc A53 (-78.075, -37.3622) -> (-74.0235, -37.109) centre (-76.1871, -35.0308) ccw projected
  line L21 (-78.075, -37.3622) -> (-83.0768, -33.3119) projected
  arc A54 (-83.4142, -27.4014) -> (-83.0768, -33.3119) centre (-80.5595, -30.2033) ccw projected
  arc A55 (-94.9045, -47.3031) -> (-94.9045, -71.9432) centre (-50.585, -59.6232) ccw projected
  arc A56 (-89.6172, -44.6401) -> (-94.9045, -47.3031) centre (-91.0507, -48.3745) ccw projected
  line L22 (-89.6172, -44.6401) -> (-83.6086, -46.9466) projected
  arc A57 (-81.8021, -50.5819) -> (-83.6086, -46.9466) centre (-84.6837, -49.7474) ccw projected
  arc A58 (-81.8021, -50.5819) -> (-81.8021, -68.6644) centre (-50.585, -59.6232) ccw projected
  arc A59 (-83.6086, -72.2997) -> (-81.8021, -68.6644) centre (-84.6837, -69.499) ccw projected
  line L23 (-83.6086, -72.2997) -> (-89.6172, -74.6062) projected
  arc A60 (-94.9045, -71.9432) -> (-89.6172, -74.6062) centre (-91.0507, -70.8719) ccw projected
  circle A61 centre (-36.0848, -126.8778) radius 16 projected
  circle A62 centre (-50.585, -59.6232) radius 8 projected
  circle A63 centre (4.8498, -18.875) radius 8 projected
  circle A64 centre (-26.0687, -154.0932) radius 1.5 projected
  circle A65 centre (-104.9663, -72.7226) radius 1.5 projected
  circle A66 centre (-102.1649, -37.0532) radius 1.5 projected
  circle A67 centre (14.3857, 5.6417) radius 1.5 projected
  circle A68 centre (13.3039, -43.7854) radius 1.5 projected
  circle A69 centre (31.1494, -18.2994) radius 1.5 projected
  circle A70 centre (-15.6668, -2.4109) radius 1.5 projected
  circle A71 centre (-91.1309, -21.0881) radius 1.5 projected
  circle A72 centre (-106.5395, -53.3794) radius 1.5 projected
  circle A73 centre (-53.3702, -150.5044) radius 1.5 projected
  circle A74 centre (-7.6073, -133.6622) radius 1.5 projected
  line L24 (-9.7265, -123.6247) -> (9.9725, -47.9268) projected
  line L25 (9.9725, -47.9268) -> (17.8509, -46.5376) projected
  line L26 (17.8509, -46.5376) -> (17.2063, -42.8816) projected
  arc A75 (17.2063, -42.8816) -> (31.6348, -22.2755) centre (4.8498, -18.875) ccw projected
  line L27 (31.6348, -22.2755) -> (35.2909, -21.6308) projected
  line L28 (35.2909, -21.6308) -> (33.9017, -13.7524) projected
  line L29 (33.9017, -13.7524) -> (27.008, -14.9679) projected
  arc A76 (27.008, -14.9679) -> (16.0998, 0.6106) centre (4.8498, -18.875) ccw projected
  line L30 (16.0998, 0.6106) -> (19.5998, 6.6727) projected
  line L31 (19.5998, 6.6727) -> (12.6716, 10.6727) projected
  line L32 (12.6716, 10.6727) -> (10.8154, 7.4577) projected
  arc A77 (10.8154, 7.4577) -> (-13.4829, 0.947) centre (4.8498, -18.875) ccw projected
  line L33 (-13.4829, 0.947) -> (-16.6979, 2.8032) projected
  line L34 (-16.6979, 2.8032) -> (-20.6979, -4.125) projected
  line L35 (-20.6979, -4.125) -> (-55.4348, -7.3477) projected
  arc A78 (-55.4348, -7.3477) -> (-76.835, -14.1568) centre (-50.585, -59.6232) ccw projected
  line L36 (-76.835, -14.1568) -> (-80.3713, -8.0318) projected
  line L37 (-80.3713, -8.0318) -> (-92.9509, -17.9357) projected
  arc A79 (-92.9509, -17.9357) -> (-96.423, -21.7867) centre (-50.585, -59.6232) ccw projected
  line L38 (-96.423, -21.7867) -> (-95.6743, -22.4047) projected
  arc A80 (-95.3624, -25.1669) -> (-95.6743, -22.4047) centre (-96.9475, -23.9472) ccw projected
  arc A81 (-95.3624, -25.1669) -> (-100.1355, -32.4754) centre (-50.585, -59.6232) ccw projected
  arc A82 (-102.79, -33.3003) -> (-100.1355, -32.4754) centre (-101.8895, -31.5145) ccw projected
  line L39 (-102.79, -33.3003) -> (-103.9829, -32.6988) projected
  arc A83 (-103.9829, -32.6988) -> (-106.5047, -38.4279) centre (-50.585, -59.6232) ccw projected
  line L40 (-106.5047, -38.4279) -> (-109.6106, -50.019) projected
  arc A84 (-109.6106, -50.019) -> (-110.2911, -56.2415) centre (-50.585, -59.6232) ccw projected
  line L41 (-110.2911, -56.2415) -> (-108.9573, -56.317) projected
  arc A85 (-107.0709, -58.3586) -> (-108.9573, -56.317) centre (-109.0704, -58.3138) ccw projected
  arc A86 (-107.0709, -58.3586) -> (-106.5915, -67.0745) centre (-50.585, -59.6232) ccw projected
  arc A87 (-108.2427, -69.3107) -> (-106.5915, -67.0745) centre (-108.5741, -67.3383) ccw projected
  line L42 (-108.2427, -69.3107) -> (-109.2001, -69.4715) projected
  arc A88 (-109.2001, -69.4715) -> (-108.1187, -74.5427) centre (-50.585, -59.6232) ccw projected
  line L43 (-108.1187, -74.5427) -> (-102.1764, -89.4094) projected
  line L44 (-102.1764, -89.4094) -> (-96.0514, -85.8732) projected
  arc A89 (-96.0514, -85.8732) -> (-93.2051, -90.2791) centre (-50.585, -59.6232) ccw projected
  line L45 (-93.2051, -90.2791) -> (-56.6733, -141.0681) projected
  arc A90 (-57.2313, -148.7428) -> (-56.6733, -141.0681) centre (-61.5442, -144.5716) ccw projected
  line L46 (-57.2313, -148.7428) -> (-59.0263, -150.5988) projected
  line L47 (-59.0263, -150.5988) -> (-54.7134, -154.77) projected
  line L48 (-54.7134, -154.77) -> (-51.8854, -154.7228) projected
  line L49 (-51.8854, -154.7228) -> (-50.3657, -153.1515) projected
  arc A91 (-48.0859, -152.7278) -> (-50.3657, -153.1515) centre (-48.9281, -154.5419) ccw projected
  arc A92 (-48.0859, -152.7278) -> (-31.6953, -155.0377) centre (-36.0848, -126.8778) ccw projected
  arc A93 (-29.5104, -156.3231) -> (-31.6953, -155.0377) centre (-31.3873, -157.0139) ccw projected
  line L50 (-29.5104, -156.3231) -> (-29.1318, -157.3516) projected
  line L51 (-29.1318, -157.3516) -> (-26.5641, -158.5378) projected
  line L52 (-26.5641, -158.5378) -> (-22.8103, -157.1563) projected
  line L53 (-22.8103, -157.1563) -> (-21.6241, -154.5886) projected
  line L54 (-21.6241, -154.5886) -> (-22.0027, -153.56) projected
  arc A94 (-21.1722, -151.1649) -> (-22.0027, -153.56) centre (-20.1257, -152.8693) ccw projected
  arc A95 (-21.1722, -151.1649) -> (-10.1895, -138.7808) centre (-36.0848, -126.8778) ccw projected
  arc A96 (-8.179, -137.6255) -> (-10.1895, -138.7808) centre (-8.3723, -139.6161) ccw projected
  line L55 (-8.179, -137.6255) -> (-6.0033, -137.8368) projected
  line L56 (-6.0033, -137.8368) -> (-3.8193, -136.0394) projected
  line L57 (-3.8193, -136.0394) -> (-3.2394, -130.0675) projected
  line L58 (-3.2394, -130.0675) -> (-5.371, -129.8605) projected
  arc A97 (-9.7265, -123.6247) -> (-5.371, -129.8605) centre (-4.8877, -124.8839) ccw projected
  line L59 (-20.6106, -30.2033) -> (-10.1194, -48.3745)
  circle A98 centre (-15.365, -39.2889) radius 2.1
  point P0 (0, 0)
  dimension "d74" = 4.2
  constraints: 2 end point, 1 centre point, 1 midpoint
  measures "d74" diameter of A98
extrude "Extrusion10" cut sketch "Sketch11" against normal blind 10 contours A98 L59 | L59 A98
pattern_circular "Circular Pattern5" count 6 over 360 about axis through (-50.585, -59.6232, 5) along (0, 0, -1) of "Extrusion9", "Extrusion10"